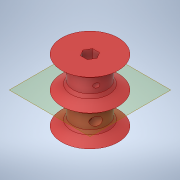
# Autodesk Inventor part: hexSpoolForArmV01
Saved by Autodesk Inventor 2022.2 (Build 262287010, 287A)
## iProperties
Created: 2019-02-24
Part Number: hexSpoolForArmV01
Material: PC/ABS Plastic
Document SubType Name: Modeling
Designer: steele
Density: 0.357273 g/cm^3
Appearance: Smooth - Red
holeForString: 0.200 in
stringDiameter: 0.120 in
clearanceForString: 0.080 in
clearanceForHexShaft: 0.040 in
spoolInteriorDiameter: 1.500 in
spoolInteriroRadius: 0.750 in
spoolExteriorDiameter: 2.500 in
spoolExteriorRadius: 1.250 in
hexHoleChamfer: 0.063 in
stringHoleCenterFromHexShaft: 0.370 in
textCircleDiameter: 1.875 in
textHeight: 0.180 in
textDepth: 0.050 in
Author: steele
Autodesk Inventor part; units mm, degrees
(part 1 of 2)
ref_plane "XZ Plane" through (0, 0, 0) normal (0, 1, 0) x (-1, 0, 0)
ref_plane "XY Plane" through (0, 0, 0) normal (0, 0, 1) x (1, 0, 0)
sketch "Sketch15" plane through (0, 0, 0) normal (0, 0, 1) x (1, 0, 0)
  line L0 (31.75, 0) -> (31.75, 69.85) construction
  line L1 (12.065, 0) -> (31.75, 0)
  line L2 (19.05, 0) -> (19.05, 69.85) construction
  line L3 (0, 69.85) -> (0, 0)
  line L4 (19.05, 17.4625) -> (31.75, 17.4625) construction
  line L5 (31.75, 0) -> (19.05, 7.3323)
  line L6 (31.75, 34.925) -> (19.05, 27.5927)
  line L7 (19.05, 27.5927) -> (31.75, 27.5927) construction
  line L8 (19.05, 27.5927) -> (19.05, 7.3323)
  line L9 (31.75, 34.925) -> (19.05, 42.2573)
  line L10 (19.05, 42.2573) -> (19.05, 62.5177)
  line L11 (19.05, 62.5177) -> (31.75, 69.85)
  line L12 (31.75, 34.925) -> (19.05, 34.925) construction
  line L13 (19.05, 62.5177) -> (31.75, 62.5177) construction
  line L14 (12.065, 0) -> (0, 0)
  line L15 (31.75, 69.85) -> (0, 69.85)
  dimension "d86" = 69.85
  dimension "d89" = 34.925
  dimension "centerLineForSpool" = 17.4625
  dimension "d93" = 30
  dimension "d94" = 30
  dimension "d95" = 30
  dimension "d96" = 30
  dimension "d156" = 31.75
  dimension "d158" = 31.75
  constraints: 32 end point, 9 point on line, 3 horizontal, 2 midpoint, 2 perpendicular, 1 collinear, 1 vertical
  measures "d86" distance of L0.start L0.end
  measures "d89" distance from line of L6.start L1
  measures "centerLineForSpool" distance from line of L4.start L1
  measures "d93" angle of L5 L1
  measures "d94" angle of L6 L7
  measures "d95" angle of L9 L12
  measures "d96" angle of L11 L13
  measures "d156" distance from line of L0.end L3
  measures "d158" distance from line of L0.start L3
revolve "Revolution2" add sketch "Sketch15" angle 360 about axis through (0, 69.85, 0) along (0, -1, 0)
sketch "Sketch16" plane through (0, 0, 0) normal (0, -1, 0) x (1, 0, 0)
  line L0 (-7.9189, 0) -> (-3.9595, 6.858)
  line L1 (-3.9595, 6.858) -> (3.9595, 6.858)
  line L2 (3.9595, 6.858) -> (7.9189, 0)
  line L3 (7.9189, 0) -> (3.9595, -6.858)
  line L4 (3.9595, -6.858) -> (-3.9595, -6.858)
  line L5 (-3.9595, -6.858) -> (-7.9189, 0)
  point P0 (0, 0)
  point P1 (0, 0)
  dimension "d103" = 13.716
  constraints: 12 end point, 1 coincident, 1 horizontal, 13 other
  measures "d103" distance between parallel lines of L1 L4
extrude "Extrusion11" cut sketch "Sketch16" against normal through all
sketch "Sketch17" plane through (0, 0, 0) normal (1, 0, 0) x (0, 1, 0)
  circle A0 centre (52.3875, 9.398) radius 2.54
  circle A1 centre (17.4625, 9.398) radius 2.54
  line L0 (0, 31.75) -> (0, -31.75) projected
  line L1 (69.85, 31.75) -> (69.85, -31.75) projected
  line L2 (0, 6.858) -> (69.85, 6.858) projected
  point P0 (0, 0)
  point P1 (72.39, 6.858)
  dimension "d110" = 17.4625
  dimension "d111" = 17.4625
  dimension "d112" = 5.08
  constraints: 2 centre point, 2 tangent, 1 equal radius
  measures "d110" distance from line of A1.centre L0
  measures "d111" distance from line of A0.centre L1
  measures "d112" diameter of A0
extrude "Extrusion13" cut sketch "Sketch17" along normal through all both and the other way through all
ref_plane "Work Plane4" through (-19.05, 0, 0) normal (1, 0, 0) x (0, 1, 0)
sketch "Sketch22" plane through (-19.05, 0, 0) normal (1, 0, 0) x (0, 1, 0)
  spline S0 degree 7 poles (54.9275, 9.398) (54.9275, 9.7003) (54.8855, 9.9947) (54.8055, 10.2759) (54.6914, 10.5396) (54.547, 10.7823) (54.3764, 11.0012) (53.983, 11.3946) (53.7559, 11.5694) (53.5066, 11.7139) (53.24, 11.8248) (52.9612, 11.9) (52.6753, 11.938) (52.1137, 11.938) (51.8403, 11.9036) (51.5721, 11.8349) (51.3141, 11.7328) (51.0711, 11.5991) (50.848, 11.4367) (50.4419, 11.0554) (50.2585, 10.8324) (50.103, 10.5833) (49.9797, 10.311) (49.8931, 10.0193) (49.8475, 9.713) (49.8475, 9.1243) (49.8819, 8.8508) (49.9506, 8.5825) (50.0528, 8.3245) (50.1864, 8.0817) (50.3487, 7.8586) (50.7502, 7.431) (50.9916, 7.2397) (51.2531, 7.0865) (51.5286, 6.9719) (51.8128, 6.8958) (52.1007, 6.858) (52.7051, 6.858) (53.0247, 6.9043) (53.3394, 6.998) (53.642, 7.1395) (53.9245, 7.3282) (54.1787, 7.563) (54.5393, 8.0279) (54.6661, 8.2331) (54.7705, 8.4538) (54.8497, 8.6855) (54.9021, 8.9235) (54.9275, 9.1626) (54.9275, 9.398) knots 0 0 0 0 0 0 0 0 0.127217 0.127217 0.127217 0.127217 0.127217 0.127217 0.25952 0.25952 0.25952 0.25952 0.25952 0.25952 0.385403 0.385403 0.385403 0.385403 0.385403 0.385403 0.516079 0.516079 0.516079 0.516079 0.516079 0.516079 0.629606 0.629606 0.629606 0.629606 0.629606 0.629606 0.75956 0.75956 0.75956 0.75956 0.75956 0.75956 0.903464 0.903464 0.903464 0.903464 0.903464 0.903464 1 1 1 1 1 1 1 1 projected
  circle A0 centre (52.3875, 9.398) radius 4.7625
  circle A1 centre (52.3875, 9.398) radius 2.54 construction
  line L0 (52.3875, 6.858) -> (17.4625, 6.858) construction
  line L1 (69.85, 31.75) -> (69.85, -31.75) construction
  point P0 (0, 0)
  point P1 (69.85, 6.858)
  point P2 (72.39, 6.858)
  dimension "d121" = 17.4625
  dimension "d122" = 5.08
  dimension "d125" = 9.525
  constraints: 2 centre point, 1 concentric, 1 tangent, 1 vertical alignment
  measures "d121" distance from line of A1.centre L1
  measures "d122" diameter of A1
  measures "d125" diameter of A0
extrude "Extrusion16" cut sketch "Sketch22" along normal blind 11.1125
ref_plane "Work Plane5" through (19.05, 0, 0) normal (1, 0, 0) x (0, 1, 0)
sketch "Sketch23" plane through (19.05, 0, 0) normal (1, 0, 0) x (0, 1, 0)
  line L0 (17.4625, 6.858) -> (52.3875, 6.858) projected
  circle A0 centre (17.4625, 9.398) radius 2.54 construction
  line L1 (0, 31.75) -> (0, -31.75) projected
  circle A1 centre (17.4625, 9.398) radius 4.7625
  point P0 (0, 0)
  dimension "d127" = 5.08
  dimension "d128" = 17.4625
  dimension "d129" = 9.525
  constraints: 2 centre point, 1 coincident, 1 tangent
  measures "d127" diameter of A0
  measures "d128" distance from line of A0.centre L1
  measures "d129" diameter of A1
extrude "Extrusion17" cut sketch "Sketch23" against normal blind 11.1125
chamfer "Chamfer12" distance 2.3813 angle 45 4 edges at (-19.05, 62.5177, 0) (-19.05, 42.2573, 0) (-19.05, 27.5927, 0) (-19.05, 7.3323, 0)
ref_plane "Work Plane6" through (0, 34.925, 0) normal (0, -1, 0) x (1, 0, 0)
sketch "Sketch26" plane through (0, 0, 0) normal (0, -1, 0) x (1, 0, 0)
  circle A0 centre (0, 0) radius 23.8125 construction
  spline S0 degree 2 poles (-24.7852, 3.5176) (-24.5019, 3.4962) (-24.0902, 3.2484) (-23.9621, 3.0591) knots 0 0 0 1 2 2 2
  spline S1 degree 2 poles (-23.9621, 3.0591) (-23.809, 2.8308) (-23.706, 2.3091) (-23.7359, 1.9119) knots 0 0 0 1 2 2 2
  line L0 (-23.7359, 1.9119) -> (-23.8505, 0.3941)
  line L1 (-23.8505, 0.3941) -> (-27.6497, 0.6808)
  line L2 (-27.6497, 0.6808) -> (-27.5486, 2.02)
  spline S2 degree 2 poles (-27.5486, 2.02) (-27.517, 2.4388) (-27.4198, 2.8649) (-27.3041, 3.045) knots 0 0 0 1 2 2 2
  spline S3 degree 2 poles (-27.3041, 3.045) (-27.1807, 3.2432) (-26.7962, 3.4154) (-26.556, 3.3973) knots 0 0 0 1 2 2 2
  spline S4 degree 2 poles (-26.556, 3.3973) (-26.2789, 3.3764) (-25.8657, 3.0665) (-25.7827, 2.8126) knots 0 0 0 1 2 2 2
  line L3 (-25.7827, 2.8126) -> (-25.7643, 2.8112)
  spline S5 degree 2 poles (-25.7643, 2.8112) (-25.6637, 3.1597) (-25.1731, 3.5468) (-24.7852, 3.5176) knots 0 0 0 1 2 2 2
  spline S6 degree 2 poles (-24.8749, 2.5335) (-25.0535, 2.547) (-25.2643, 2.4205) (-25.3273, 2.2828) knots 0 0 0 1 2 2 2
  spline S7 degree 2 poles (-25.3273, 2.2828) (-25.3677, 2.1992) (-25.3968, 1.8948) (-25.4159, 1.6424) knots 0 0 0 1 2 2 2
  line L4 (-25.4159, 1.6424) -> (-25.4291, 1.4669)
  line L5 (-25.4291, 1.4669) -> (-24.4716, 1.3946)
  line L6 (-24.4716, 1.3946) -> (-24.4677, 1.447)
  spline S8 degree 2 poles (-24.4677, 1.447) (-24.4398, 1.8164) (-24.4277, 2.1004) (-24.4812, 2.253) knots 0 0 0 1 2 2 2
  spline S9 degree 2 poles (-24.4812, 2.253) (-24.5299, 2.3867) (-24.7364, 2.5231) (-24.8749, 2.5335) knots 0 0 0 1 2 2 2
  spline S10 degree 2 poles (-26.4414, 2.4133) (-26.5338, 2.4203) (-26.7349, 2.3395) (-26.7855, 2.2442) knots 0 0 0 1 2 2 2
  spline S11 degree 2 poles (-26.7855, 2.2442) (-26.8355, 2.1551) (-26.8612, 1.897) (-26.8805, 1.6414) knots 0 0 0 1 2 2 2
  line L7 (-26.8805, 1.6414) -> (-26.8854, 1.5768)
  line L8 (-26.8854, 1.5768) -> (-26.0787, 1.5159)
  line L9 (-26.0787, 1.5159) -> (-26.0697, 1.636)
  spline S12 degree 2 poles (-26.0697, 1.636) (-26.0513, 1.8792) (-26.0457, 2.0769) (-26.0871, 2.1853) knots 0 0 0 1 2 2 2
  spline S13 degree 2 poles (-26.0871, 2.1853) (-26.1339, 2.3034) (-26.3152, 2.4038) (-26.4414, 2.4133) knots 0 0 0 1 2 2 2
  spline S14 degree 2 poles (-24.3269, 6.9191) (-23.6337, 6.7652) (-23.0058, 5.832) (-23.159, 5.1418) knots 0 0 0 1 2 2 2
  spline S15 degree 2 poles (-23.159, 5.1418) (-23.3116, 4.4545) (-24.2766, 3.8686) (-24.9698, 4.0224) knots 0 0 0 1 2 2 2
  spline S16 degree 2 poles (-24.9698, 4.0224) (-25.6691, 4.1776) (-26.2926, 5.1162) (-26.1401, 5.8034) knots 0 0 0 1 2 2 2
  spline S17 degree 2 poles (-26.1401, 5.8034) (-25.9875, 6.4906) (-25.0232, 7.0736) (-24.3269, 6.9191) knots 0 0 0 1 2 2 2
  spline S18 degree 2 poles (-24.5196, 6.0225) (-24.7698, 6.078) (-25.1224, 6.0709) (-25.2379, 6.0207) knots 0 0 0 1 2 2 2
  spline S19 degree 2 poles (-25.2379, 6.0207) (-25.3608, 5.9657) (-25.4857, 5.7878) (-25.5131, 5.6643) knots 0 0 0 1 2 2 2
  spline S20 degree 2 poles (-25.5131, 5.6643) (-25.5399, 5.5437) (-25.5097, 5.3377) (-25.4246, 5.2366) knots 0 0 0 1 2 2 2
  spline S21 degree 2 poles (-25.4246, 5.2366) (-25.3449, 5.1399) (-25.0243, 4.9738) (-24.7651, 4.9163) knots 0 0 0 1 2 2 2
  spline S22 degree 2 poles (-24.7651, 4.9163) (-24.5089, 4.8594) (-24.1737, 4.8736) (-24.0618, 4.9215) knots 0 0 0 1 2 2 2
  spline S23 degree 2 poles (-24.0618, 4.9215) (-23.95, 4.9694) (-23.8127, 5.1604) (-23.7846, 5.287) knots 0 0 0 1 2 2 2
  spline S24 degree 2 poles (-23.7846, 5.287) (-23.7612, 5.3924) (-23.8035, 5.6295) (-23.8792, 5.7159) knots 0 0 0 1 2 2 2
  spline S25 degree 2 poles (-23.8792, 5.7159) (-23.968, 5.8147) (-24.2543, 5.9636) (-24.5196, 6.0225) knots 0 0 0 1 2 2 2
  spline S26 degree 2 poles (-22.3455, 8.0742) (-22.5236, 7.5576) (-23.1127, 7.2315) (-23.5973, 7.3985) knots 0 0 0 1 2 2 2
  line L10 (-23.5973, 7.3985) -> (-24.8671, 7.8361)
  line L11 (-24.8671, 7.8361) -> (-24.9787, 7.5121)
  line L12 (-24.9787, 7.5121) -> (-25.5684, 7.7153)
  line L13 (-25.5684, 7.7153) -> (-25.4567, 8.0393)
  line L14 (-25.4567, 8.0393) -> (-26.2332, 8.3069)
  line L15 (-26.2332, 8.3069) -> (-25.9415, 9.1534)
  line L16 (-25.9415, 9.1534) -> (-25.165, 8.8858)
  line L17 (-25.165, 8.8858) -> (-24.8834, 9.7031)
  line L18 (-24.8834, 9.7031) -> (-24.2937, 9.4999)
  line L19 (-24.2937, 9.4999) -> (-24.5754, 8.6826)
  line L20 (-24.5754, 8.6826) -> (-23.6092, 8.3497)
  spline S27 degree 2 poles (-23.6092, 8.3497) (-23.4661, 8.3004) (-23.251, 8.2328) (-23.1543, 8.2386) knots 0 0 0 1 2 2 2
  spline S28 degree 2 poles (-23.1543, 8.2386) (-23.0576, 8.2445) (-22.899, 8.3825) (-22.8426, 8.546) knots 0 0 0 1 2 2 2
  spline S29 degree 2 poles (-22.8426, 8.546) (-22.8185, 8.616) (-22.8014, 8.8551) (-22.8097, 8.9069) knots 0 0 0 1 2 2 2
  line L21 (-22.8097, 8.9069) -> (-22.7846, 8.9799)
  line L22 (-22.7846, 8.9799) -> (-22.1891, 8.7747)
  spline S30 degree 2 poles (-22.1891, 8.7747) (-22.2013, 8.6254) (-22.2671, 8.3019) (-22.3455, 8.0742) knots 0 0 0 1 2 2 2
  spline S31 degree 2 poles (-21.5159, 10.0789) (-21.7403, 9.5806) (-22.3567, 9.3097) (-22.824, 9.5202) knots 0 0 0 1 2 2 2
  line L23 (-22.824, 9.5202) -> (-24.0486, 10.0718)
  line L24 (-24.0486, 10.0718) -> (-24.1894, 9.7593)
  line L25 (-24.1894, 9.7593) -> (-24.758, 10.0154)
  line L26 (-24.758, 10.0154) -> (-24.6173, 10.3279)
  line L27 (-24.6173, 10.3279) -> (-25.3661, 10.6652)
  line L28 (-25.3661, 10.6652) -> (-24.9984, 11.4816)
  line L29 (-24.9984, 11.4816) -> (-24.2495, 11.1443)
  line L30 (-24.2495, 11.1443) -> (-23.8945, 11.9325)
  line L31 (-23.8945, 11.9325) -> (-23.3259, 11.6764)
  line L32 (-23.3259, 11.6764) -> (-23.6809, 10.8882)
  line L33 (-23.6809, 10.8882) -> (-22.7491, 10.4685)
  spline S32 degree 2 poles (-22.7491, 10.4685) (-22.6111, 10.4063) (-22.4031, 10.3194) (-22.3062, 10.3164) knots 0 0 0 1 2 2 2
  spline S33 degree 2 poles (-22.3062, 10.3164) (-22.2094, 10.3134) (-22.0389, 10.4364) (-21.9679, 10.594) knots 0 0 0 1 2 2 2
  spline S34 degree 2 poles (-21.9679, 10.594) (-21.9374, 10.6616) (-21.8986, 10.8981) (-21.9021, 10.9505) knots 0 0 0 1 2 2 2
  line L34 (-21.9021, 10.9505) -> (-21.8704, 11.0208)
  line L35 (-21.8704, 11.0208) -> (-21.2961, 10.7622)
  spline S35 degree 2 poles (-21.2961, 10.7622) (-21.322, 10.6147) (-21.4169, 10.2985) (-21.5159, 10.0789) knots 0 0 0 1 2 2 2
  spline S36 degree 2 poles (-20.9405, 14.1834) (-20.3302, 13.8203) (-20.0259, 12.7376) (-20.3873, 12.1299) knots 0 0 0 1 2 2 2
  spline S37 degree 2 poles (-20.3873, 12.1299) (-20.7473, 11.5249) (-21.8471, 11.2703) (-22.4574, 11.6334) knots 0 0 0 1 2 2 2
  spline S38 degree 2 poles (-22.4574, 11.6334) (-23.0731, 11.9996) (-23.3716, 13.0861) (-23.0117, 13.6911) knots 0 0 0 1 2 2 2
  spline S39 degree 2 poles (-23.0117, 13.6911) (-22.6518, 14.2961) (-21.5534, 14.548) (-20.9405, 14.1834) knots 0 0 0 1 2 2 2
  spline S40 degree 2 poles (-21.404, 13.3921) (-21.6242, 13.5232) (-21.9614, 13.6267) (-22.0868, 13.6151) knots 0 0 0 1 2 2 2
  spline S41 degree 2 poles (-22.0868, 13.6151) (-22.2208, 13.6014) (-22.395, 13.4715) (-22.4597, 13.3627) knots 0 0 0 1 2 2 2
  spline S42 degree 2 poles (-22.4597, 13.3627) (-22.5229, 13.2566) (-22.5586, 13.0516) (-22.5095, 12.9289) knots 0 0 0 1 2 2 2
  spline S43 degree 2 poles (-22.5095, 12.9289) (-22.464, 12.812) (-22.2115, 12.5541) (-21.9833, 12.4183) knots 0 0 0 1 2 2 2
  spline S44 degree 2 poles (-21.9833, 12.4183) (-21.7578, 12.2841) (-21.435, 12.1927) (-21.3137, 12.2032) knots 0 0 0 1 2 2 2
  spline S45 degree 2 poles (-21.3137, 12.2032) (-21.1925, 12.2137) (-21.0024, 12.3521) (-20.9361, 12.4636) knots 0 0 0 1 2 2 2
  spline S46 degree 2 poles (-20.9361, 12.4636) (-20.8809, 12.5564) (-20.8468, 12.7948) (-20.8917, 12.9006) knots 0 0 0 1 2 2 2
  spline S47 degree 2 poles (-20.8917, 12.9006) (-20.9451, 13.0222) (-21.1705, 13.2532) (-21.404, 13.3921) knots 0 0 0 1 2 2 2
  line L36 (-17.2449, 16.4705) -> (-18.3346, 17.4051)
  spline S48 degree 2 poles (-18.3346, 17.4051) (-18.4963, 17.5438) (-18.7267, 17.7211) (-18.8211, 17.7532) knots 0 0 0 1 2 2 2
  spline S49 degree 2 poles (-18.8211, 17.7532) (-18.9176, 17.7831) (-19.0854, 17.7155) (-19.1798, 17.6053) knots 0 0 0 1 2 2 2
  spline S50 degree 2 poles (-19.1798, 17.6053) (-19.2462, 17.528) (-19.3068, 17.3197) (-19.3199, 17.1764) knots 0 0 0 1 2 2 2
  line L37 (-19.3199, 17.1764) -> (-17.7755, 15.8518)
  line L38 (-17.7755, 15.8518) -> (-18.3624, 15.1674)
  line L39 (-18.3624, 15.1674) -> (-19.4522, 16.1021)
  spline S51 degree 2 poles (-19.4522, 16.1021) (-19.6116, 16.2388) (-19.8463, 16.4157) (-19.9407, 16.4479) knots 0 0 0 1 2 2 2
  spline S52 degree 2 poles (-19.9407, 16.4479) (-20.0372, 16.4777) (-20.205, 16.4101) (-20.2994, 16.2999) knots 0 0 0 1 2 2 2
  spline S53 degree 2 poles (-20.2994, 16.2999) (-20.3698, 16.2179) (-20.4311, 15.9899) (-20.4416, 15.8686) knots 0 0 0 1 2 2 2
  line L40 (-20.4416, 15.8686) -> (-18.8971, 14.544)
  line L41 (-18.8971, 14.544) -> (-19.48, 13.8644)
  line L42 (-19.48, 13.8644) -> (-21.6619, 15.7357)
  line L43 (-21.6619, 15.7357) -> (-21.079, 16.4154)
  line L44 (-21.079, 16.4154) -> (-20.8376, 16.2083)
  spline S54 degree 2 poles (-20.8376, 16.2083) (-20.8355, 16.4953) (-20.7396, 16.9297) (-20.5808, 17.1148) knots 0 0 0 1 2 2 2
  spline S55 degree 2 poles (-20.5808, 17.1148) (-20.41, 17.314) (-19.9588, 17.4559) (-19.7007, 17.3727) knots 0 0 0 1 2 2 2
  spline S56 degree 2 poles (-19.7007, 17.3727) (-19.7166, 17.724) (-19.616, 18.2397) (-19.4632, 18.4179) knots 0 0 0 1 2 2 2
  spline S57 degree 2 poles (-19.4632, 18.4179) (-19.3326, 18.5702) (-19.0294, 18.7292) (-18.8607, 18.7268) knots 0 0 0 1 2 2 2
  spline S58 degree 2 poles (-18.8607, 18.7268) (-18.6768, 18.7277) (-18.3102, 18.5719) (-18.0781, 18.3729) knots 0 0 0 1 2 2 2
  line L45 (-18.0781, 18.3729) -> (-16.6579, 17.1548)
  line L46 (-16.6579, 17.1548) -> (-17.2449, 16.4705)
  line L47 (-12.3046, 20.4503) -> (-13.0897, 19.9027)
  line L48 (-13.0897, 19.9027) -> (-14.0558, 21.2879)
  line L49 (-14.0558, 21.2879) -> (-15.122, 20.5443)
  line L50 (-15.122, 20.5443) -> (-14.1558, 19.1591)
  line L51 (-14.1558, 19.1591) -> (-14.9408, 18.6115)
  line L52 (-14.9408, 18.6115) -> (-17.1205, 21.7365)
  line L53 (-17.1205, 21.7365) -> (-16.3354, 22.284)
  line L54 (-16.3354, 22.284) -> (-15.537, 21.1394)
  line L55 (-15.537, 21.1394) -> (-14.4709, 21.883)
  line L56 (-14.4709, 21.883) -> (-15.2693, 23.0277)
  line L57 (-15.2693, 23.0277) -> (-14.4843, 23.5752)
  line L58 (-14.4843, 23.5752) -> (-12.3046, 20.4503)
  spline S59 degree 2 poles (-10.3027, 21.3842) (-11.0331, 21.0225) (-12.1559, 21.3346) (-12.4752, 21.9792) knots 0 0 0 1 2 2 2
  spline S60 degree 2 poles (-12.4752, 21.9792) (-12.7877, 22.61) (-12.4356, 23.7216) (-11.7826, 24.0451) knots 0 0 0 1 2 2 2
  spline S61 degree 2 poles (-11.7826, 24.0451) (-11.1933, 24.337) (-10.2791, 23.9939) (-9.9859, 23.4018) knots 0 0 0 1 2 2 2
  line L59 (-9.9859, 23.4018) -> (-9.842, 23.1113)
  line L60 (-9.842, 23.1113) -> (-11.6044, 22.2383)
  spline S62 degree 2 poles (-11.6044, 22.2383) (-11.5042, 22.064) (-11.2563, 21.8904) (-11.1156, 21.8706) knots 0 0 0 1 2 2 2
  spline S63 degree 2 poles (-11.1156, 21.8706) (-10.9776, 21.8493) (-10.6708, 21.9255) (-10.5075, 22.0064) knots 0 0 0 1 2 2 2
  spline S64 degree 2 poles (-10.5075, 22.0064) (-10.3692, 22.0749) (-10.1282, 22.2701) (-10.0408, 22.3788) knots 0 0 0 1 2 2 2
  spline S65 degree 2 poles (-10.0408, 22.3788) (-9.9617, 22.4697) (-9.8464, 22.6542) (-9.8131, 22.719) knots 0 0 0 1 2 2 2
  line L61 (-9.8131, 22.719) -> (-9.7273, 22.7615)
  line L62 (-9.7273, 22.7615) -> (-9.3984, 22.0975)
  spline S66 degree 2 poles (-9.3984, 22.0975) (-9.4788, 22.0094) (-9.6064, 21.8635) (-9.7338, 21.7591) knots 0 0 0 1 2 2 2
  spline S67 degree 2 poles (-9.7338, 21.7591) (-9.846, 21.6587) (-10.1035, 21.4829) (-10.3027, 21.3842) knots 0 0 0 1 2 2 2
  spline S68 degree 2 poles (-10.8731, 23.2035) (-11.0047, 23.4553) (-11.3617, 23.6127) (-11.5914, 23.4989) knots 0 0 0 1 2 2 2
  spline S69 degree 2 poles (-11.5914, 23.4989) (-11.8265, 23.3824) (-11.9524, 22.9687) (-11.847, 22.7211) knots 0 0 0 1 2 2 2
  line L63 (-11.847, 22.7211) -> (-10.8731, 23.2035)
  line L64 (-6.1681, 23.0543) -> (-7.1619, 22.7162)
  line L65 (-7.1619, 22.7162) -> (-7.9447, 23.3207)
  line L66 (-7.9447, 23.3207) -> (-8.2113, 22.3593)
  line L67 (-8.2113, 22.3593) -> (-9.1847, 22.0283)
  line L68 (-9.1847, 22.0283) -> (-8.6453, 23.7314)
  line L69 (-8.6453, 23.7314) -> (-10.0927, 24.7556)
  line L70 (-10.0927, 24.7556) -> (-9.0989, 25.0936)
  line L71 (-9.0989, 25.0936) -> (-8.3298, 24.5008)
  line L72 (-8.3298, 24.5008) -> (-8.0787, 25.4406)
  line L73 (-8.0787, 25.4406) -> (-7.1053, 25.7717)
  line L74 (-7.1053, 25.7717) -> (-7.6351, 24.0979)
  line L75 (-7.6351, 24.0979) -> (-6.1681, 23.0543)
  line L76 (-4.7798, 23.3323) -> (-5.6624, 23.1339)
  line L77 (-5.6624, 23.1339) -> (-5.8832, 24.1159)
  line L78 (-5.8832, 24.1159) -> (-5.0006, 24.3143)
  line L79 (-5.0006, 24.3143) -> (-4.7798, 23.3323)
  line L80 (-5.1895, 25.1547) -> (-6.0721, 24.9563)
  line L81 (-6.0721, 24.9563) -> (-6.2929, 25.9383)
  line L82 (-6.2929, 25.9383) -> (-5.4103, 26.1368)
  line L83 (-5.4103, 26.1368) -> (-5.1895, 25.1547)
  spline S70 degree 2 poles (0.2628, 25.758) (0.2859, 25.2646) (0.1633, 24.517) (-0.0008, 24.259) knots 0 0 0 1 2 2 2
  spline S71 degree 2 poles (-0.0008, 24.259) (-0.1619, 24.0041) (-0.7083, 23.7251) (-1.1092, 23.7063) knots 0 0 0 1 2 2 2
  spline S72 degree 2 poles (-1.1092, 23.7063) (-1.5133, 23.6874) (-2.0803, 23.9142) (-2.2679, 24.1589) knots 0 0 0 1 2 2 2
  spline S73 degree 2 poles (-2.2679, 24.1589) (-2.4554, 24.4005) (-2.6471, 25.1271) (-2.6702, 25.6206) knots 0 0 0 1 2 2 2
  spline S74 degree 2 poles (-2.6702, 25.6206) (-2.6939, 26.1264) (-2.5701, 26.8493) (-2.4034, 27.1167) knots 0 0 0 1 2 2 2
  spline S75 degree 2 poles (-2.4034, 27.1167) (-2.2364, 27.378) (-1.6835, 27.6512) (-1.2949, 27.6694) knots 0 0 0 1 2 2 2
  spline S76 degree 2 poles (-1.2949, 27.6694) (-0.8848, 27.6886) (-0.3236, 27.4553) (-0.1358, 27.2075) knots 0 0 0 1 2 2 2
  spline S77 degree 2 poles (-0.1358, 27.2075) (0.0486, 26.9658) (0.2404, 26.2361) (0.2628, 25.758) knots 0 0 0 1 2 2 2
  spline S78 degree 2 poles (-0.6964, 25.7131) (-0.7295, 26.4194) (-0.9875, 26.9791) (-1.262, 26.9662) knots 0 0 0 1 2 2 2
  spline S79 degree 2 poles (-1.262, 26.9662) (-1.5365, 26.9534) (-1.7441, 26.3718) (-1.7109, 25.6625) knots 0 0 0 1 2 2 2
  spline S80 degree 2 poles (-1.7109, 25.6625) (-1.6782, 24.9654) (-1.4167, 24.3966) (-1.1422, 24.4095) knots 0 0 0 1 2 2 2
  spline S81 degree 2 poles (-1.1422, 24.4095) (-0.8708, 24.4222) (-0.6636, 25.013) (-0.6964, 25.7131) knots 0 0 0 1 2 2 2
  line L84 (1.8183, 23.7473) -> (0.9151, 23.7992)
  line L85 (0.9151, 23.7992) -> (0.973, 24.8041)
  line L86 (0.973, 24.8041) -> (1.8761, 24.7521)
  line L87 (1.8761, 24.7521) -> (1.8183, 23.7473)
  spline S82 degree 2 poles (5.4564, 24.5447) (5.4082, 24.2491) (5.1255, 23.7822) (4.8981, 23.6347) knots 0 0 0 1 2 2 2
  spline S83 degree 2 poles (4.8981, 23.6347) (4.6707, 23.4873) (4.096, 23.3777) (3.6998, 23.4424) knots 0 0 0 1 2 2 2
  spline S84 degree 2 poles (3.6998, 23.4424) (3.2798, 23.5141) (2.6988, 23.7497) (2.5152, 23.8704) knots 0 0 0 1 2 2 2
  line L88 (2.5152, 23.8704) -> (2.649, 24.6901)
  line L89 (2.649, 24.6901) -> (2.7343, 24.6761)
  spline S85 degree 2 poles (2.7343, 24.6761) (2.801, 24.6246) (2.9608, 24.4921) (3.0951, 24.4139) knots 0 0 0 1 2 2 2
  spline S86 degree 2 poles (3.0951, 24.4139) (3.2207, 24.3402) (3.4866, 24.2249) (3.6541, 24.1975) knots 0 0 0 1 2 2 2
  spline S87 degree 2 poles (3.6541, 24.1975) (3.8004, 24.1736) (4.1536, 24.1911) (4.2732, 24.2717) knots 0 0 0 1 2 2 2
  spline S88 degree 2 poles (4.2732, 24.2717) (4.3618, 24.3354) (4.4774, 24.5074) (4.5028, 24.6628) knots 0 0 0 1 2 2 2
  spline S89 degree 2 poles (4.5028, 24.6628) (4.5247, 24.7969) (4.4458, 25.0037) (4.3669, 25.076) knots 0 0 0 1 2 2 2
  spline S90 degree 2 poles (4.3669, 25.076) (4.2529, 25.1822) (3.8951, 25.2907) (3.7641, 25.312) knots 0 0 0 1 2 2 2
  spline S91 degree 2 poles (3.7641, 25.312) (3.5569, 25.3459) (3.1529, 25.343) (3.0037, 25.3298) knots 0 0 0 1 2 2 2
  line L90 (3.0037, 25.3298) -> (2.9214, 25.3432)
  line L91 (2.9214, 25.3432) -> (3.2661, 27.4549)
  line L92 (3.2661, 27.4549) -> (5.7587, 27.0481)
  line L93 (5.7587, 27.0481) -> (5.6428, 26.3381)
  line L94 (5.6428, 26.3381) -> (4.043, 26.5992)
  line L95 (4.043, 26.5992) -> (3.9411, 25.9745)
  spline S92 degree 2 poles (3.9411, 25.9745) (4.0183, 25.9682) (4.2295, 25.94) (4.2874, 25.9305) knots 0 0 0 1 2 2 2
  spline S93 degree 2 poles (4.2874, 25.9305) (4.5586, 25.8862) (4.9978, 25.7019) (5.1592, 25.5598) knots 0 0 0 1 2 2 2
  spline S94 degree 2 poles (5.1592, 25.5598) (5.3496, 25.3849) (5.5112, 24.8798) (5.4564, 24.5447) knots 0 0 0 1 2 2 2
  line L96 (8.834, 23.121) -> (8.3417, 23.2742)
  line L97 (8.3417, 23.2742) -> (8.0747, 22.4163)
  line L98 (8.0747, 22.4163) -> (7.1932, 22.6907)
  line L99 (7.1932, 22.6907) -> (7.4602, 23.5486)
  line L100 (7.4602, 23.5486) -> (5.8565, 24.0477)
  line L101 (5.8565, 24.0477) -> (6.0675, 24.7258)
  line L102 (6.0675, 24.7258) -> (8.2987, 26.3466)
  line L103 (8.2987, 26.3466) -> (9.2097, 26.0631)
  line L104 (9.2097, 26.0631) -> (8.5454, 23.9287)
  line L105 (8.5454, 23.9287) -> (9.0377, 23.7755)
  line L106 (9.0377, 23.7755) -> (8.834, 23.121)
  line L107 (7.6639, 24.203) -> (8.0493, 25.4412)
  line L108 (8.0493, 25.4412) -> (6.7412, 24.4902)
  line L109 (6.7412, 24.4902) -> (7.6639, 24.203)
  spline S95 degree 2 poles (12.3202, 22.6221) (12.109, 22.1755) (11.6499, 21.5729) (11.3839, 21.422) knots 0 0 0 1 2 2 2
  spline S96 degree 2 poles (11.3839, 21.422) (11.122, 21.2726) (10.5086, 21.2826) (10.1457, 21.4542) knots 0 0 0 1 2 2 2
  spline S97 degree 2 poles (10.1457, 21.4542) (9.7801, 21.6271) (9.3859, 22.0935) (9.335, 22.3976) knots 0 0 0 1 2 2 2
  spline S98 degree 2 poles (9.335, 22.3976) (9.2828, 22.6989) (9.4546, 23.4306) (9.6657, 23.8772) knots 0 0 0 1 2 2 2
  spline S99 degree 2 poles (9.6657, 23.8772) (9.8822, 24.3349) (10.3307, 24.9152) (10.6034, 25.0731) knots 0 0 0 1 2 2 2
  spline S100 degree 2 poles (10.6034, 25.0731) (10.8736, 25.2254) (11.4899, 25.2072) (11.8416, 25.0409) knots 0 0 0 1 2 2 2
  spline S101 degree 2 poles (11.8416, 25.0409) (12.2129, 24.8654) (12.5988, 24.396) (12.6484, 24.0891) knots 0 0 0 1 2 2 2
  spline S102 degree 2 poles (12.6484, 24.0891) (12.6978, 23.7891) (12.5247, 23.0547) (12.3202, 22.6221) knots 0 0 0 1 2 2 2
  spline S103 degree 2 poles (11.4521, 23.0325) (11.7543, 23.6717) (11.7891, 24.2871) (11.5407, 24.4045) knots 0 0 0 1 2 2 2
  spline S104 degree 2 poles (11.5407, 24.4045) (11.2923, 24.522) (10.836, 24.1059) (10.5325, 23.4639) knots 0 0 0 1 2 2 2
  spline S105 degree 2 poles (10.5325, 23.4639) (10.2342, 22.8331) (10.1982, 22.2081) (10.4466, 22.0906) knots 0 0 0 1 2 2 2
  spline S106 degree 2 poles (10.4466, 22.0906) (10.6923, 21.9745) (11.1525, 22.3989) (11.4521, 23.0325) knots 0 0 0 1 2 2 2
  line L110 (14.8417, 18.6496) -> (13.1842, 19.8561)
  line L111 (13.1842, 19.8561) -> (13.5748, 20.3928)
  line L112 (13.5748, 20.3928) -> (14.0167, 20.0712)
  line L113 (14.0167, 20.0712) -> (15.4775, 22.0782)
  line L114 (15.4775, 22.0782) -> (15.0356, 22.3998)
  line L115 (15.0356, 22.3998) -> (15.4263, 22.9365)
  line L116 (15.4263, 22.9365) -> (17.0838, 21.7301)
  line L117 (17.0838, 21.7301) -> (16.6932, 21.1934)
  line L118 (16.6932, 21.1934) -> (16.2513, 21.515)
  line L119 (16.2513, 21.515) -> (14.7905, 19.5079)
  line L120 (14.7905, 19.5079) -> (15.2324, 19.1863)
  line L121 (15.2324, 19.1863) -> (14.8417, 18.6496)
  spline S107 degree 2 poles (19.1212, 17.2884) (18.7512, 16.9032) (17.8332, 16.6206) (17.421, 16.7041) knots 0 0 0 1 2 2 2
  spline S108 degree 2 poles (17.421, 16.7041) (17.0746, 16.7714) (16.4944, 17.1747) (16.2117, 17.4463) knots 0 0 0 1 2 2 2
  line L122 (16.2117, 17.4463) -> (15.3522, 18.272)
  line L123 (15.3522, 18.272) -> (17.9919, 21.0195)
  line L124 (17.9919, 21.0195) -> (18.8424, 20.2023)
  spline S109 degree 2 poles (18.8424, 20.2023) (19.1318, 19.9243) (19.5666, 19.3652) (19.6524, 19.0088) knots 0 0 0 1 2 2 2
  spline S110 degree 2 poles (19.6524, 19.0088) (19.7549, 18.5763) (19.5041, 17.6869) (19.1212, 17.2884) knots 0 0 0 1 2 2 2
  spline S111 degree 2 poles (18.4175, 17.9731) (18.6785, 18.2447) (18.8637, 18.8118) (18.777, 19.1048) knots 0 0 0 1 2 2 2
  spline S112 degree 2 poles (18.777, 19.1048) (18.7095, 19.3153) (18.4172, 19.6261) (18.2035, 19.8314) knots 0 0 0 1 2 2 2
  line L125 (18.2035, 19.8314) -> (18.1901, 19.8443)
  line L126 (18.1901, 19.8443) -> (16.5366, 18.1232)
  line L127 (16.5366, 18.1232) -> (16.5499, 18.1104)
  spline S113 degree 2 poles (16.5499, 18.1104) (16.7815, 17.8879) (17.1148, 17.5976) (17.3473, 17.5499) knots 0 0 0 1 2 2 2
  spline S114 degree 2 poles (17.3473, 17.5499) (17.6191, 17.4942) (18.1565, 17.7014) (18.4175, 17.9731) knots 0 0 0 1 2 2 2
  line L128 (18.7665, 14.6649) -> (18.196, 15.3669)
  line L129 (18.196, 15.3669) -> (18.9772, 16.0017)
  line L130 (18.9772, 16.0017) -> (19.5477, 15.2996)
  line L131 (19.5477, 15.2996) -> (18.7665, 14.6649)
  line L132 (20.2162, 15.8429) -> (19.6457, 16.5449)
  line L133 (19.6457, 16.5449) -> (20.4268, 17.1797)
  line L134 (20.4268, 17.1797) -> (20.9973, 16.4776)
  line L135 (20.9973, 16.4776) -> (20.2162, 15.8429)
  line L136 (21.4602, 10.4073) -> (20.236, 12.6058)
  line L137 (20.236, 12.6058) -> (20.816, 12.9287)
  line L138 (20.816, 12.9287) -> (21.2065, 12.2274)
  line L139 (21.2065, 12.2274) -> (22.968, 13.2082)
  line L140 (22.968, 13.2082) -> (22.5774, 13.9096)
  line L141 (22.5774, 13.9096) -> (23.1196, 14.2115)
  spline S115 degree 2 poles (23.1196, 14.2115) (23.2053, 14.0577) (23.4155, 13.7754) (23.5097, 13.7078) knots 0 0 0 1 2 2 2
  spline S116 degree 2 poles (23.5097, 13.7078) (23.6222, 13.6326) (23.869, 13.6145) (24.0099, 13.6789) knots 0 0 0 1 2 2 2
  line L142 (24.0099, 13.6789) -> (24.4155, 12.9505)
  line L143 (24.4155, 12.9505) -> (21.6586, 11.4154)
  line L144 (21.6586, 11.4154) -> (22.0402, 10.7302)
  line L145 (22.0402, 10.7302) -> (21.4602, 10.4073)
  line L146 (22.0748, 8.941) -> (21.7194, 9.7729)
  line L147 (21.7194, 9.7729) -> (22.645, 10.1684)
  line L148 (22.645, 10.1684) -> (23.0004, 9.3365)
  line L149 (23.0004, 9.3365) -> (22.0748, 8.941)
  spline S117 degree 2 poles (24.4081, 6.0379) (24.122, 5.9496) (23.578, 5.9949) (23.3448, 6.133) knots 0 0 0 1 2 2 2
  spline S118 degree 2 poles (23.3448, 6.133) (23.1115, 6.271) (22.7576, 6.7369) (22.6392, 7.1204) knots 0 0 0 1 2 2 2
  spline S119 degree 2 poles (22.6392, 7.1204) (22.5165, 7.5284) (22.4689, 8.1535) (22.4952, 8.3717) knots 0 0 0 1 2 2 2
  line L150 (22.4952, 8.3717) -> (23.2888, 8.6167)
  line L151 (23.2888, 8.6167) -> (23.3143, 8.5341)
  spline S120 degree 2 poles (23.3143, 8.5341) (23.2978, 8.4515) (23.2504, 8.2494) (23.2401, 8.0944) knots 0 0 0 1 2 2 2
  spline S121 degree 2 poles (23.2401, 8.0944) (23.23, 7.9491) (23.245, 7.6597) (23.2951, 7.4974) knots 0 0 0 1 2 2 2
  spline S122 degree 2 poles (23.2951, 7.4974) (23.3388, 7.3558) (23.5116, 7.0472) (23.637, 6.9761) knots 0 0 0 1 2 2 2
  spline S123 degree 2 poles (23.637, 6.9761) (23.7335, 6.9251) (23.939, 6.8981) (24.0895, 6.9445) knots 0 0 0 1 2 2 2
  spline S124 degree 2 poles (24.0895, 6.9445) (24.2193, 6.9846) (24.3694, 7.1473) (24.399, 7.2501) knots 0 0 0 1 2 2 2
  spline S125 degree 2 poles (24.399, 7.2501) (24.4434, 7.3995) (24.3813, 7.7681) (24.3421, 7.895) knots 0 0 0 1 2 2 2
  spline S126 degree 2 poles (24.3421, 7.895) (24.2802, 8.0956) (24.0978, 8.4561) (24.0196, 8.5838) knots 0 0 0 1 2 2 2
  line L152 (24.0196, 8.5838) -> (23.995, 8.6635)
  line L153 (23.995, 8.6635) -> (26.0394, 9.2947)
  line L154 (26.0394, 9.2947) -> (26.7844, 6.8815)
  line L155 (26.7844, 6.8815) -> (26.0971, 6.6692)
  line L156 (26.0971, 6.6692) -> (25.6189, 8.2181)
  line L157 (25.6189, 8.2181) -> (25.0141, 8.0313)
  spline S127 degree 2 poles (25.0141, 8.0313) (25.0428, 7.9594) (25.1115, 7.7577) (25.1288, 7.7016) knots 0 0 0 1 2 2 2
  spline S128 degree 2 poles (25.1288, 7.7016) (25.2099, 7.4391) (25.2403, 6.9638) (25.1849, 6.756) knots 0 0 0 1 2 2 2
  spline S129 degree 2 poles (25.1849, 6.756) (25.113, 6.5076) (24.7326, 6.1381) (24.4081, 6.0379) knots 0 0 0 1 2 2 2
  line L158 (27.5311, 3.9195) -> (26.0206, 3.808)
  line L159 (26.0206, 3.808) -> (25.9288, 4.3248)
  line L160 (25.9288, 4.3248) -> (27.3853, 4.7402)
  line L161 (27.3853, 4.7402) -> (27.5311, 3.9195)
  line L162 (27.3427, 4.9804) -> (25.8322, 4.869)
  line L163 (25.8322, 4.869) -> (25.7404, 5.3858)
  line L164 (25.7404, 5.3858) -> (27.197, 5.8012)
  line L165 (27.197, 5.8012) -> (27.3427, 4.9804)
  spline S130 degree 2 poles (25.6584, -2.5378) (24.7325, -2.5129) (23.7005, -1.4966) (23.7236, -0.6386) knots 0 0 0 1 2 2 2
  spline S131 degree 2 poles (23.7236, -0.6386) (23.7469, 0.2225) (24.8443, 1.1751) (25.7579, 1.1504) knots 0 0 0 1 2 2 2
  spline S132 degree 2 poles (25.7579, 1.1504) (26.6746, 1.1257) (27.716, 0.1154) (27.6927, -0.7457) knots 0 0 0 1 2 2 2
  spline S133 degree 2 poles (27.6927, -0.7457) (27.6696, -1.6037) (26.5812, -2.5627) (25.6584, -2.5378) knots 0 0 0 1 2 2 2
  spline S134 degree 2 poles (25.685, -1.5502) (26.0276, -1.5594) (26.5098, -1.4335) (26.6642, -1.3172) knots 0 0 0 1 2 2 2
  spline S135 degree 2 poles (26.6642, -1.3172) (26.8249, -1.201) (26.969, -0.8961) (26.9735, -0.7294) knots 0 0 0 1 2 2 2
  spline S136 degree 2 poles (26.9735, -0.7294) (26.9783, -0.5535) (26.8595, -0.263) (26.7026, -0.126) knots 0 0 0 1 2 2 2
  spline S137 degree 2 poles (26.7026, -0.126) (26.5576, -0.0047) (26.0708, 0.1536) (25.7313, 0.1628) knots 0 0 0 1 2 2 2
  spline S138 degree 2 poles (25.7313, 0.1628) (25.3794, 0.1723) (24.9127, 0.0459) (24.752, -0.0703) knots 0 0 0 1 2 2 2
  spline S139 degree 2 poles (24.752, -0.0703) (24.5914, -0.1864) (24.4472, -0.4944) (24.4427, -0.6611) knots 0 0 0 1 2 2 2
  spline S140 degree 2 poles (24.4427, -0.6611) (24.4381, -0.8309) (24.5747, -1.1496) (24.7259, -1.268) knots 0 0 0 1 2 2 2
  spline S141 degree 2 poles (24.7259, -1.268) (24.8892, -1.3959) (25.327, -1.5405) (25.685, -1.5502) knots 0 0 0 1 2 2 2
  spline S142 degree 2 poles (24.8787, -6.7497) (24.3547, -6.6464) (23.6209, -6.0266) (23.4684, -5.6346) knots 0 0 0 1 2 2 2
  spline S143 degree 2 poles (23.4684, -5.6346) (23.3379, -5.3068) (23.3638, -4.6007) (23.4397, -4.216) knots 0 0 0 1 2 2 2
  line L166 (23.4397, -4.216) -> (23.6702, -3.0467)
  line L167 (23.6702, -3.0467) -> (27.4082, -3.7836)
  line L168 (27.4082, -3.7836) -> (27.1801, -4.9407)
  spline S144 degree 2 poles (27.1801, -4.9407) (27.1025, -5.3345) (26.867, -6.0025) (26.6134, -6.2672) knots 0 0 0 1 2 2 2
  spline S145 degree 2 poles (26.6134, -6.2672) (26.3049, -6.5871) (25.421, -6.8566) (24.8787, -6.7497) knots 0 0 0 1 2 2 2
  spline S146 degree 2 poles (25.0747, -5.7876) (25.4442, -5.8605) (26.0215, -5.7099) (26.2213, -5.4787) knots 0 0 0 1 2 2 2
  spline S147 degree 2 poles (26.2213, -5.4787) (26.3619, -5.3081) (26.4655, -4.8943) (26.5228, -4.6035) knots 0 0 0 1 2 2 2
  line L169 (26.5228, -4.6035) -> (26.5264, -4.5853)
  line L170 (26.5264, -4.5853) -> (24.1848, -4.1237)
  line L171 (24.1848, -4.1237) -> (24.1812, -4.1419)
  spline S148 degree 2 poles (24.1812, -4.1419) (24.1191, -4.4569) (24.0549, -4.8943) (24.1403, -5.1157) knots 0 0 0 1 2 2 2
  spline S149 degree 2 poles (24.1403, -5.1157) (24.2403, -5.3745) (24.7051, -5.7148) (25.0747, -5.7876) knots 0 0 0 1 2 2 2
  line L172 (24.2539, -8.4521) -> (24.5365, -7.5927)
  line L173 (24.5365, -7.5927) -> (25.4927, -7.9071)
  line L174 (25.4927, -7.9071) -> (25.2101, -8.7665)
  line L175 (25.2101, -8.7665) -> (24.2539, -8.4521)
  line L176 (22.4794, -7.8687) -> (22.762, -7.0093)
  line L177 (22.762, -7.0093) -> (23.7182, -7.3237)
  line L178 (23.7182, -7.3237) -> (23.4356, -8.183)
  line L179 (23.4356, -8.183) -> (22.4794, -7.8687)
  line L180 (20.2719, -12.5853) -> (21.5946, -10.117)
  line L181 (21.5946, -10.117) -> (22.1416, -10.4101)
  spline S150 degree 2 poles (22.1416, -10.4101) (22.2243, -10.8573) (22.3968, -11.5943) (22.4948, -11.8885) knots 0 0 0 1 2 2 2
  spline S151 degree 2 poles (22.4948, -11.8885) (22.6206, -12.2747) (22.8971, -12.7066) (23.1039, -12.8174) knots 0 0 0 1 2 2 2
  spline S152 degree 2 poles (23.1039, -12.8174) (23.338, -12.9428) (23.7386, -12.7967) (23.8727, -12.5463) knots 0 0 0 1 2 2 2
  spline S153 degree 2 poles (23.8727, -12.5463) (23.9413, -12.4184) (24.0012, -12.1563) (24.0149, -12.013) knots 0 0 0 1 2 2 2
  spline S154 degree 2 poles (24.0149, -12.013) (24.0244, -11.871) (24.0031, -11.6494) (23.9978, -11.594) knots 0 0 0 1 2 2 2
  line L182 (23.9978, -11.594) -> (24.0328, -11.5287)
  line L183 (24.0328, -11.5287) -> (24.7648, -11.921)
  spline S155 degree 2 poles (24.7648, -11.921) (24.757, -12.099) (24.5748, -12.7789) (24.4245, -13.0592) knots 0 0 0 1 2 2 2
  spline S156 degree 2 poles (24.4245, -13.0592) (24.1037, -13.6579) (23.2407, -13.9871) (22.759, -13.729) knots 0 0 0 1 2 2 2
  spline S157 degree 2 poles (22.759, -13.729) (22.4624, -13.57) (22.0411, -12.9835) (21.8881, -12.4846) knots 0 0 0 1 2 2 2
  spline S158 degree 2 poles (21.8881, -12.4846) (21.7961, -12.1726) (21.6888, -11.6212) (21.6687, -11.5018) knots 0 0 0 1 2 2 2
  line L184 (21.6687, -11.5018) -> (20.9059, -12.9251)
  line L185 (20.9059, -12.9251) -> (20.2719, -12.5853)
  line L186 (19.4503, -13.745) -> (19.9583, -12.9965)
  line L187 (19.9583, -12.9965) -> (20.7911, -13.5617)
  line L188 (20.7911, -13.5617) -> (20.2831, -14.3102)
  line L189 (20.2831, -14.3102) -> (19.4503, -13.745)
  line L190 (19.6138, -18.4158) -> (18.3284, -15.2034)
  line L191 (18.3284, -15.2034) -> (19.0131, -14.3915)
  line L192 (19.0131, -14.3915) -> (20.279, -17.6844)
  line L193 (20.279, -17.6844) -> (21.4494, -16.2965)
  line L194 (21.4494, -16.2965) -> (21.9993, -16.7603)
  line L195 (21.9993, -16.7603) -> (20.1921, -18.9034)
  line L196 (20.1921, -18.9034) -> (19.6138, -18.4158)
  spline S159 degree 2 poles (15.6797, -19.656) (15.4799, -19.4329) (15.294, -18.9197) (15.322, -18.6502) knots 0 0 0 1 2 2 2
  spline S160 degree 2 poles (15.322, -18.6502) (15.35, -18.3806) (15.6255, -17.8644) (15.9245, -17.5967) knots 0 0 0 1 2 2 2
  spline S161 degree 2 poles (15.9245, -17.5967) (16.244, -17.3148) (16.7921, -17.0105) (17.0014, -16.9433) knots 0 0 0 1 2 2 2
  line L197 (17.0014, -16.9433) -> (17.5554, -17.562)
  line L198 (17.5554, -17.562) -> (17.491, -17.6197)
  spline S162 degree 2 poles (17.491, -17.6197) (17.409, -17.6392) (17.2056, -17.6805) (17.0604, -17.7359) knots 0 0 0 1 2 2 2
  spline S163 degree 2 poles (17.0604, -17.7359) (16.9242, -17.7874) (16.6675, -17.9219) (16.541, -18.0352) knots 0 0 0 1 2 2 2
  spline S164 degree 2 poles (16.541, -18.0352) (16.4306, -18.1341) (16.2224, -18.42) (16.2101, -18.5636) knots 0 0 0 1 2 2 2
  spline S165 degree 2 poles (16.2101, -18.5636) (16.2041, -18.6726) (16.2653, -18.8706) (16.3704, -18.9879) knots 0 0 0 1 2 2 2
  spline S166 degree 2 poles (16.3704, -18.9879) (16.461, -19.0891) (16.6715, -19.1575) (16.7773, -19.1415) knots 0 0 0 1 2 2 2
  spline S167 degree 2 poles (16.7773, -19.1415) (16.9316, -19.1194) (17.2406, -18.9091) (17.3395, -18.8205) knots 0 0 0 1 2 2 2
  spline S168 degree 2 poles (17.3395, -18.8205) (17.4959, -18.6804) (17.7473, -18.3641) (17.8307, -18.2397) knots 0 0 0 1 2 2 2
  line L199 (17.8307, -18.2397) -> (17.8928, -18.1841)
  line L200 (17.8928, -18.1841) -> (19.3201, -19.7781)
  line L201 (19.3201, -19.7781) -> (17.4386, -21.4629)
  line L202 (17.4386, -21.4629) -> (16.9587, -20.927)
  line L203 (16.9587, -20.927) -> (18.1663, -19.8457)
  line L204 (18.1663, -19.8457) -> (17.7441, -19.3741)
  spline S169 degree 2 poles (17.7441, -19.3741) (17.6907, -19.4302) (17.5361, -19.5769) (17.4924, -19.6161) knots 0 0 0 1 2 2 2
  spline S170 degree 2 poles (17.4924, -19.6161) (17.2877, -19.7994) (16.8685, -20.0255) (16.6566, -20.0619) knots 0 0 0 1 2 2 2
  spline S171 degree 2 poles (16.6566, -20.0619) (16.4008, -20.1003) (15.9063, -19.909) (15.6797, -19.656) knots 0 0 0 1 2 2 2
  line L205 (15.0591, -23.3783) -> (14.327, -22.0524)
  line L206 (14.327, -22.0524) -> (14.7583, -21.7532)
  line L207 (14.7583, -21.7532) -> (15.744, -22.9031)
  line L208 (15.744, -22.9031) -> (15.0591, -23.3783)
  line L209 (15.9444, -22.7641) -> (15.2123, -21.4382)
  line L210 (15.2123, -21.4382) -> (15.6436, -21.139)
  line L211 (15.6436, -21.139) -> (16.6293, -22.2889)
  line L212 (16.6293, -22.2889) -> (15.9444, -22.7641)
  line L213 (7.8943, -22.5233) -> (8.7742, -22.1466)
  line L214 (8.7742, -22.1466) -> (9.4388, -23.6992)
  line L215 (9.4388, -23.6992) -> (10.6338, -23.1876)
  line L216 (10.6338, -23.1876) -> (9.9691, -21.635)
  line L217 (9.9691, -21.635) -> (10.849, -21.2583)
  line L218 (10.849, -21.2583) -> (12.3485, -24.7609)
  line L219 (12.3485, -24.7609) -> (11.4686, -25.1376)
  line L220 (11.4686, -25.1376) -> (10.9193, -23.8546)
  line L221 (10.9193, -23.8546) -> (9.7244, -24.3662)
  line L222 (9.7244, -24.3662) -> (10.2736, -25.6491)
  line L223 (10.2736, -25.6491) -> (9.3937, -26.0258)
  line L224 (9.3937, -26.0258) -> (7.8943, -22.5233)
  spline S172 degree 2 poles (6.1095, -22.9606) (6.6355, -22.8123) (7.2393, -23.1103) (7.3784, -23.6036) knots 0 0 0 1 2 2 2
  line L225 (7.3784, -23.6036) -> (7.743, -24.8962)
  line L226 (7.743, -24.8962) -> (8.0729, -24.8032)
  line L227 (8.0729, -24.8032) -> (8.2422, -25.4034)
  line L228 (8.2422, -25.4034) -> (7.9124, -25.4965)
  line L229 (7.9124, -25.4965) -> (8.1353, -26.2869)
  line L230 (8.1353, -26.2869) -> (7.2736, -26.53)
  line L231 (7.2736, -26.53) -> (7.0506, -25.7396)
  line L232 (7.0506, -25.7396) -> (6.2186, -25.9743)
  line L233 (6.2186, -25.9743) -> (6.0492, -25.374)
  line L234 (6.0492, -25.374) -> (6.8813, -25.1393)
  line L235 (6.8813, -25.1393) -> (6.6038, -24.1557)
  spline S173 degree 2 poles (6.6038, -24.1557) (6.5628, -24.0101) (6.4956, -23.7949) (6.4357, -23.7187) knots 0 0 0 1 2 2 2
  spline S174 degree 2 poles (6.4357, -23.7187) (6.3757, -23.6426) (6.1719, -23.5911) (6.0055, -23.638) knots 0 0 0 1 2 2 2
  spline S175 degree 2 poles (6.0055, -23.638) (5.9341, -23.6581) (5.728, -23.7804) (5.6902, -23.8168) knots 0 0 0 1 2 2 2
  line L236 (5.6902, -23.8168) -> (5.6159, -23.8377)
  line L237 (5.6159, -23.8377) -> (5.4449, -23.2315)
  spline S176 degree 2 poles (5.4449, -23.2315) (5.5745, -23.1565) (5.8777, -23.026) (6.1095, -22.9606) knots 0 0 0 1 2 2 2
  line L238 (4.3879, -25.3069) -> (5.2764, -25.1366)
  line L239 (5.2764, -25.1366) -> (5.4659, -26.1251)
  line L240 (5.4659, -26.1251) -> (4.5774, -26.2954)
  line L241 (4.5774, -26.2954) -> (4.3879, -25.3069)
  line L242 (4.0363, -23.4723) -> (4.9248, -23.302)
  line L243 (4.9248, -23.302) -> (5.1143, -24.2906)
  line L244 (5.1143, -24.2906) -> (4.2258, -24.4608)
  line L245 (4.2258, -24.4608) -> (4.0363, -23.4723)
  spline S177 degree 2 poles (-1.0458, -24.9858) (-1.05, -24.7049) (-0.8501, -24.2418) (-0.6519, -24.0782) knots 0 0 0 1 2 2 2
  spline S178 degree 2 poles (-0.6519, -24.0782) (-0.4536, -23.9147) (0.0902, -23.7336) (0.4823, -23.7277) knots 0 0 0 1 2 2 2
  spline S179 degree 2 poles (0.4823, -23.7277) (0.9268, -23.721) (1.565, -23.8596) (1.7671, -23.9492) knots 0 0 0 1 2 2 2
  line L246 (1.7671, -23.9492) -> (1.7795, -24.7765)
  line L247 (1.7795, -24.7765) -> (1.6869, -24.7779)
  spline S180 degree 2 poles (1.6869, -24.7779) (1.475, -24.6483) (0.9071, -24.4593) (0.6725, -24.4628) knots 0 0 0 1 2 2 2
  spline S181 degree 2 poles (0.6725, -24.4628) (0.5335, -24.4649) (0.2101, -24.5192) (0.1002, -24.6011) knots 0 0 0 1 2 2 2
  spline S182 degree 2 poles (0.1002, -24.6011) (0.0147, -24.6672) (-0.0874, -24.8571) (-0.0848, -25.0269) knots 0 0 0 1 2 2 2
  spline S183 degree 2 poles (-0.0848, -25.0269) (-0.0823, -25.1967) (0.0686, -25.3766) (0.1928, -25.418) knots 0 0 0 1 2 2 2
  spline S184 degree 2 poles (0.1928, -25.418) (0.3169, -25.4594) (0.6597, -25.4635) (0.7925, -25.4615) knots 0 0 0 1 2 2 2
  line L248 (0.7925, -25.4615) -> (0.9561, -25.459)
  line L249 (0.9561, -25.459) -> (0.9662, -26.1289)
  line L250 (0.9662, -26.1289) -> (0.8149, -26.1312)
  spline S185 degree 2 poles (0.8149, -26.1312) (0.642, -26.1338) (0.3492, -26.1691) (0.248, -26.2169) knots 0 0 0 1 2 2 2
  spline S186 degree 2 poles (0.248, -26.2169) (0.1469, -26.2678) (0.0353, -26.4424) (0.0375, -26.5906) knots 0 0 0 1 2 2 2
  spline S187 degree 2 poles (0.0375, -26.5906) (0.0393, -26.7079) (0.1495, -26.8514) (0.2273, -26.8904) knots 0 0 0 1 2 2 2
  spline S188 degree 2 poles (0.2273, -26.8904) (0.3206, -26.9353) (0.568, -26.9624) (0.6545, -26.9611) knots 0 0 0 1 2 2 2
  spline S189 degree 2 poles (0.6545, -26.9611) (0.7934, -26.9591) (1.0857, -26.8898) (1.2208, -26.8353) knots 0 0 0 1 2 2 2
  spline S190 degree 2 poles (1.2208, -26.8353) (1.3282, -26.7935) (1.5609, -26.6603) (1.6159, -26.6255) knots 0 0 0 1 2 2 2
  line L251 (1.6159, -26.6255) -> (1.6962, -26.6243)
  line L252 (1.6962, -26.6243) -> (1.7085, -27.4393)
  spline S191 degree 2 poles (1.7085, -27.4393) (1.5121, -27.5257) (0.8477, -27.6932) (0.4988, -27.6984) knots 0 0 0 1 2 2 2
  spline S192 degree 2 poles (0.4988, -27.6984) (0.1593, -27.7035) (-0.3426, -27.5937) (-0.5203, -27.4822) knots 0 0 0 1 2 2 2
  spline S193 degree 2 poles (-0.5203, -27.4822) (-0.7166, -27.3647) (-0.9167, -26.9972) (-0.9202, -26.7656) knots 0 0 0 1 2 2 2
  spline S194 degree 2 poles (-0.9202, -26.7656) (-0.9251, -26.4384) (-0.5558, -25.9449) (-0.2482, -25.8693) knots 0 0 0 1 2 2 2
  line L253 (-0.2482, -25.8693) -> (-0.2487, -25.8322)
  spline S195 degree 2 poles (-0.2487, -25.8322) (-0.3848, -25.8158) (-0.6457, -25.7209) (-0.7708, -25.6116) knots 0 0 0 1 2 2 2
  spline S196 degree 2 poles (-0.7708, -25.6116) (-0.8865, -25.5145) (-1.0425, -25.2019) (-1.0458, -24.9858) knots 0 0 0 1 2 2 2
  line L254 (-2.5716, -23.6775) -> (-1.6706, -23.7582)
  line L255 (-1.6706, -23.7582) -> (-1.7603, -24.7607)
  line L256 (-1.7603, -24.7607) -> (-2.6614, -24.68)
  line L257 (-2.6614, -24.68) -> (-2.5716, -23.6775)
  spline S197 degree 2 poles (-6.3878, -24.9548) (-6.2928, -24.47) (-5.9957, -23.7731) (-5.7749, -23.5616) knots 0 0 0 1 2 2 2
  spline S198 degree 2 poles (-5.7749, -23.5616) (-5.5578, -23.3524) (-4.9606, -23.2115) (-4.5668, -23.2887) knots 0 0 0 1 2 2 2
  spline S199 degree 2 poles (-4.5668, -23.2887) (-4.1699, -23.3665) (-3.6732, -23.7219) (-3.5492, -24.0042) knots 0 0 0 1 2 2 2
  spline S200 degree 2 poles (-3.5492, -24.0042) (-3.4246, -24.2834) (-3.4114, -25.0348) (-3.5064, -25.5196) knots 0 0 0 1 2 2 2
  spline S201 degree 2 poles (-3.5064, -25.5196) (-3.6039, -26.0165) (-3.8962, -26.6891) (-4.1218, -26.9092) knots 0 0 0 1 2 2 2
  spline S202 degree 2 poles (-4.1218, -26.9092) (-4.3462, -27.1232) (-4.9482, -27.2569) (-5.33, -27.1821) knots 0 0 0 1 2 2 2
  spline S203 degree 2 poles (-5.33, -27.1821) (-5.7329, -27.1031) (-6.2224, -26.7428) (-6.3458, -26.4575) knots 0 0 0 1 2 2 2
  spline S204 degree 2 poles (-6.3458, -26.4575) (-6.4673, -26.1788) (-6.4799, -25.4244) (-6.3878, -24.9548) knots 0 0 0 1 2 2 2
  spline S205 degree 2 poles (-5.4456, -25.1395) (-5.5816, -25.8333) (-5.4642, -26.4384) (-5.1945, -26.4912) knots 0 0 0 1 2 2 2
  spline S206 degree 2 poles (-5.1945, -26.4912) (-4.9249, -26.5441) (-4.5847, -26.0287) (-4.4481, -25.3319) knots 0 0 0 1 2 2 2
  spline S207 degree 2 poles (-4.4481, -25.3319) (-4.3139, -24.6471) (-4.4325, -24.0324) (-4.7022, -23.9795) knots 0 0 0 1 2 2 2
  spline S208 degree 2 poles (-4.7022, -23.9795) (-4.9688, -23.9272) (-5.3107, -24.4517) (-5.4456, -25.1395) knots 0 0 0 1 2 2 2
  line L258 (-8.5538, -26.4435) -> (-7.937, -25.0602)
  line L259 (-7.937, -25.0602) -> (-7.4384, -25.224)
  line L260 (-7.4384, -25.224) -> (-7.7618, -26.7036)
  line L261 (-7.7618, -26.7036) -> (-8.5538, -26.4435)
  line L262 (-9.5776, -26.1073) -> (-8.9608, -24.724)
  line L263 (-8.9608, -24.724) -> (-8.4621, -24.8878)
  line L264 (-8.4621, -24.8878) -> (-8.7855, -26.3674)
  line L265 (-8.7855, -26.3674) -> (-9.5776, -26.1073)
  line L266 (-15.0562, -23.2258) -> (-12.0504, -20.5435)
  line L267 (-12.0504, -20.5435) -> (-11.1806, -21.0314)
  line L268 (-11.1806, -21.0314) -> (-11.903, -24.9947)
  line L269 (-11.903, -24.9947) -> (-12.7673, -24.5098)
  line L270 (-12.7673, -24.5098) -> (-12.2273, -21.8496)
  line L271 (-12.2273, -21.8496) -> (-14.2133, -23.6986)
  line L272 (-14.2133, -23.6986) -> (-15.0562, -23.2258)
  spline S209 degree 2 poles (-18.0871, -18.3413) (-17.7608, -17.9703) (-17.1532, -17.5179) (-16.8559, -17.4464) knots 0 0 0 1 2 2 2
  spline S210 degree 2 poles (-16.8559, -17.4464) (-16.5629, -17.3751) (-15.9761, -17.554) (-15.6747, -17.8191) knots 0 0 0 1 2 2 2
  spline S211 degree 2 poles (-15.6747, -17.8191) (-15.371, -18.0863) (-15.1209, -18.6434) (-15.156, -18.9497) knots 0 0 0 1 2 2 2
  spline S212 degree 2 poles (-15.156, -18.9497) (-15.189, -19.2538) (-15.5561, -19.9095) (-15.8823, -20.2805) knots 0 0 0 1 2 2 2
  spline S213 degree 2 poles (-15.8823, -20.2805) (-16.2167, -20.6607) (-16.808, -21.0945) (-17.1138, -21.171) knots 0 0 0 1 2 2 2
  spline S214 degree 2 poles (-17.1138, -21.171) (-17.4155, -21.2428) (-18.0029, -21.0552) (-18.295, -20.7982) knots 0 0 0 1 2 2 2
  spline S215 degree 2 poles (-18.295, -20.7982) (-18.6033, -20.527) (-18.8447, -19.9693) (-18.8076, -19.6607) knots 0 0 0 1 2 2 2
  spline S216 degree 2 poles (-18.8076, -19.6607) (-18.7723, -19.3587) (-18.4032, -18.7006) (-18.0871, -18.3413) knots 0 0 0 1 2 2 2
  spline S217 degree 2 poles (-17.3661, -18.9754) (-17.833, -19.5063) (-18.0364, -20.0882) (-17.8301, -20.2696) knots 0 0 0 1 2 2 2
  spline S218 degree 2 poles (-17.8301, -20.2696) (-17.6237, -20.4511) (-17.0703, -20.1772) (-16.6013, -19.644) knots 0 0 0 1 2 2 2
  spline S219 degree 2 poles (-16.6013, -19.644) (-16.1405, -19.12) (-15.9333, -18.5292) (-16.1396, -18.3477) knots 0 0 0 1 2 2 2
  spline S220 degree 2 poles (-16.1396, -18.3477) (-16.3437, -18.1683) (-16.9032, -18.4492) (-17.3661, -18.9754) knots 0 0 0 1 2 2 2
  spline S221 degree 2 poles (-20.5979, -15.8155) (-20.2302, -15.4997) (-19.4696, -15.1438) (-19.0945, -15.1351) knots 0 0 0 1 2 2 2
  spline S222 degree 2 poles (-19.0945, -15.1351) (-18.7111, -15.1314) (-17.9975, -15.4791) (-17.6515, -15.882) knots 0 0 0 1 2 2 2
  spline S223 degree 2 poles (-17.6515, -15.882) (-17.5349, -16.0179) (-17.3166, -16.3432) (-17.2884, -16.4045) knots 0 0 0 1 2 2 2
  line L273 (-17.2884, -16.4045) -> (-17.8553, -16.8912)
  line L274 (-17.8553, -16.8912) -> (-17.9036, -16.835)
  spline S224 degree 2 poles (-17.9036, -16.835) (-17.9217, -16.757) (-18.0338, -16.5032) (-18.1846, -16.3275) knots 0 0 0 1 2 2 2
  spline S225 degree 2 poles (-18.1846, -16.3275) (-18.3073, -16.1846) (-18.6096, -15.9843) (-18.772, -15.961) knots 0 0 0 1 2 2 2
  spline S226 degree 2 poles (-18.772, -15.961) (-18.9452, -15.9347) (-19.3131, -16.0227) (-19.5253, -16.1642) knots 0 0 0 1 2 2 2